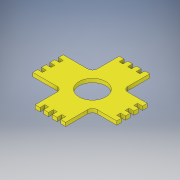
# Autodesk Inventor part: cross
Saved by Autodesk Inventor 2019.1 (Build 231200000, 200)
## iProperties
Created: 2018-10-29
Part Number: cross
Material: Generic
Document SubType Name: Modeling
Designer: kfortuna
Density: 1 g/cm^3
Appearance: Default
Author: kfortuna
Autodesk Inventor part; units mm, degrees
ref_plane "YZ Plane" through (0, 0, 0) normal (1, 0, 0) x (0, 1, 0)
ref_plane "XZ Plane" through (0, 0, 0) normal (0, 1, 0) x (-1, 0, 0)
ref_plane "XY Plane" through (0, 0, 0) normal (0, 0, 1) x (1, 0, 0)
sketch "Sketch2" plane through (0, 0, 0) normal (0, 1, 0) x (-1, 0, 0)
  line L0 (35.4299, 28.2779) -> (35.4299, 34.5151)
  line L1 (35.4299, 51.0151) -> (35.4299, 60.0151)
  line L2 (47.4299, 49.0151) -> (37.4299, 49.0151)
  line L3 (20.9299, 49.0151) -> (12.9299, 49.0151)
  line L4 (22.9299, 55.7744) -> (22.9299, 51.0151)
  line L5 (22.9299, 34.5151) -> (22.9299, 26.5151)
  line L6 (12.9299, 36.5151) -> (20.9299, 36.5151)
  line L7 (37.4299, 36.5151) -> (47.4299, 36.5151)
  line L8 (12.9299, 38.5151) -> (14.9299, 38.5151)
  line L9 (14.9299, 38.5151) -> (14.9299, 40.0151)
  line L10 (14.9299, 40.0151) -> (12.9299, 40.0151)
  line L11 (12.9299, 42.0151) -> (14.9299, 42.0151)
  line L12 (14.9299, 42.0151) -> (14.9299, 43.5151)
  line L13 (14.9299, 43.5151) -> (12.9299, 43.5151)
  line L14 (12.9299, 45.5151) -> (14.9299, 45.5151)
  line L15 (14.9299, 45.5151) -> (14.9299, 47.0151)
  line L16 (14.9299, 47.0151) -> (12.9299, 47.0151)
  line L17 (12.9299, 49.0151) -> (12.9299, 47.0151)
  line L18 (12.9299, 45.5151) -> (12.9299, 43.5151)
  line L19 (12.9299, 42.0151) -> (12.9299, 40.0151)
  line L20 (12.9299, 38.5151) -> (12.9299, 36.5151)
  line L21 (33.4299, 27.5151) -> (33.4299, 25.5151)
  line L22 (31.9299, 25.5151) -> (31.9299, 27.5151)
  line L23 (29.9299, 27.5151) -> (29.9299, 25.5151)
  line L24 (28.4299, 25.5151) -> (28.4299, 27.5151)
  line L25 (26.4299, 27.5151) -> (26.4299, 25.5151)
  line L26 (24.9299, 25.5151) -> (24.9299, 27.5151)
  line L27 (47.4299, 47.0151) -> (45.4299, 47.0151)
  line L28 (47.4299, 45.5151) -> (45.4299, 45.5151)
  line L29 (47.4299, 43.5151) -> (45.4299, 43.5151)
  line L30 (47.4299, 42.0151) -> (45.4299, 42.0151)
  line L31 (47.4299, 40.0151) -> (45.4299, 40.0151)
  line L32 (47.4299, 38.5151) -> (45.4299, 38.5151)
  line L33 (45.4299, 38.5151) -> (45.4299, 40.0151)
  line L34 (45.4299, 42.0151) -> (45.4299, 43.5151)
  line L35 (45.4299, 45.5151) -> (45.4299, 47.0151)
  line L36 (47.4299, 36.5151) -> (47.4299, 38.5151)
  line L37 (47.4299, 40.0151) -> (47.4299, 42.0151)
  line L38 (47.4299, 43.5151) -> (47.4299, 45.5151)
  line L39 (47.4299, 47.0151) -> (47.4299, 49.0151)
  line L40 (33.4299, 60.0151) -> (33.4299, 58.0151)
  line L41 (31.9299, 60.0151) -> (31.9299, 58.0151)
  line L42 (29.9299, 60.0151) -> (29.9299, 58.0151)
  line L43 (28.4299, 60.0151) -> (28.4299, 58.0151)
  line L44 (26.4299, 60.0151) -> (26.4299, 58.0151)
  line L45 (24.9299, 60.0151) -> (24.9299, 58.0151)
  arc A0 (35.4299, 51.0151) -> (37.4299, 49.0151) centre (37.4299, 51.0151) ccw
  arc A1 (37.4299, 36.5151) -> (35.4299, 34.5151) centre (37.4299, 34.5151) ccw
  arc A2 (22.9299, 34.5151) -> (20.9299, 36.5151) centre (20.9299, 34.5151) ccw
  arc A3 (20.9299, 49.0151) -> (22.9299, 51.0151) centre (20.9299, 51.0151) ccw
  line L46 (35.4299, 28.2779) -> (35.4299, 25.5151)
  line L47 (22.9299, 26.5151) -> (22.9299, 25.5151)
  line L48 (35.4299, 25.5151) -> (33.4299, 25.5151)
  line L49 (31.9299, 25.5151) -> (29.9299, 25.5151)
  line L50 (28.4299, 25.5151) -> (26.4299, 25.5151)
  line L51 (24.9299, 25.5151) -> (22.9299, 25.5151)
  line L52 (24.9299, 27.5151) -> (26.4299, 27.5151)
  line L53 (28.4299, 27.5151) -> (29.9299, 27.5151)
  line L54 (31.9299, 27.5151) -> (33.4299, 27.5151)
  line L55 (22.9299, 55.7744) -> (22.9299, 60.0151)
  line L56 (35.4299, 60.0151) -> (33.4299, 60.0151)
  line L57 (31.9299, 60.0151) -> (29.9299, 60.0151)
  line L58 (28.4299, 60.0151) -> (26.4299, 60.0151)
  line L59 (24.9299, 60.0151) -> (22.9299, 60.0151)
  line L60 (24.9299, 58.0151) -> (26.4299, 58.0151)
  line L61 (28.4299, 58.0151) -> (29.9299, 58.0151)
  line L62 (31.9299, 58.0151) -> (33.4299, 58.0151)
  circle A4 centre (29.1799, 42.7651) radius 5.5
  point P0 (0, 0)
  point P1 (35.4299, 36.5151)
  point P2 (35.4299, 49.0151)
  point P3 (22.9299, 49.0151)
  point P4 (22.9299, 36.5151)
  dimension "d25" = 1.5
  dimension "d26" = 1.5
  dimension "d27" = 1.5
  dimension "d28" = 2
  dimension "d29" = 2
  dimension "d30" = 2
  dimension "d31" = 2
  dimension "d43" = 2
  dimension "d44" = 2
  dimension "d45" = 2
  dimension "d46" = 2
  dimension "d47" = 2
  dimension "d48" = 2
  dimension "d49" = 2
  dimension "d50" = 2
  dimension "d51" = 2
  dimension "d52" = 2
  dimension "d53" = 2
  dimension "d60" = 2
  dimension "d61" = 1.5
  dimension "d62" = 1.5
  dimension "d63" = 1.5
  dimension "d64" = 1.5
  dimension "d65" = 1.5
  dimension "d66" = 1.5
  dimension "d67" = 1.5
  dimension "d68" = 1.5
  dimension "d69" = 1.5
  dimension "d70" = 2
  dimension "d71" = 2
  dimension "d72" = 2
  dimension "d74" = 2
  dimension "d75" = 2
  dimension "d76" = 2
  dimension "d77" = 2
  dimension "d78" = 2
  dimension "d79" = 2
  dimension "d80" = 2
  dimension "d81" = 11
  dimension "d82" = 11
  dimension "d83" = 11
  dimension "d84" = 11
  dimension "d85" = 2
  dimension "d86" = 2
  dimension "d87" = 2
  dimension "d88" = 2
  dimension "d89" = 10
  dimension "d90" = 10
  dimension "d91" = 12
  dimension "d92" = 12
  dimension "d97" = 2
  dimension "d98" = 2
  dimension "d99" = 2
  dimension "d100" = 8
  dimension "d102" = 2
  dimension "d105" = 6.25
  dimension "d106" = 6.25
  dimension "d109" = 2
  dimension "d110" = 0
  dimension "d111" = 2
  dimension "d112" = 0
  dimension "d113" = 2
  constraints: 126 end point, 31 parallel, 28 perpendicular, 12 horizontal, 12 point on line, 10 collinear, 8 point on circle, 8 tangent, 6 vertical, 5 centre point, 3 equal radius
  measures "d25" distance of L8.end L9.end
  measures "d26" distance of L11.end L12.end
  measures "d27" distance of L14.end L15.end
  measures "d28" distance between parallel lines of L16 L3
  measures "d29" distance between parallel lines of L13 L14
  measures "d30" distance between parallel lines of L10 L11
  measures "d31" distance between parallel lines of L6 L8
  measures "d43" distance of L8.start L8.end
  measures "d44" distance of L9.end L10.end
  measures "d45" distance of L12.end L13.end
  measures "d46" distance of L15.end L16.end
  measures "d47" distance of L32.start L32.end
  measures "d48" distance of L31.start L31.end
  measures "d49" distance of L30.start L30.end
  measures "d50" distance of L29.start L29.end
  measures "d51" distance of L28.start L28.end
  measures "d52" distance of L27.start L27.end
  measures "d53" distance from line of L27.end L2
  measures "d60" radius of A0
  measures "d61" distance of L22.end L21.start
  measures "d62" distance of L24.end L23.start
  measures "d63" distance of L26.end L25.start
  measures "d64" distance of L32.end L31.end
  measures "d65" distance of L30.end L29.end
  measures "d66" distance of L28.end L27.end
  measures "d67" distance of L41.end L40.end
  measures "d68" distance of L43.end L42.end
  measures "d69" distance of L45.end L44.end
  measures "d70" distance of L7.end L32.start
  measures "d71" distance of L31.start L30.start
  measures "d72" distance of L29.start L28.start
  measures "d74" distance of L41.start L42.start
  measures "d75" distance of L43.start L44.start
  measures "d76" distance of L45.start L55.end
  measures "d77" distance of L46.end L21.end
  measures "d78" distance of L22.start L23.end
  measures "d79" distance of L24.start L25.end
  measures "d80" distance of L26.start L47.end
  measures "d81" distance between parallel lines of L7 L48
  measures "d82" distance between parallel lines of L51 L6
  measures "d83" distance between parallel lines of L59 L3
  measures "d84" distance between parallel lines of L56 L2
  measures "d85" distance between parallel lines of L54 L48
  measures "d86" distance of L23.start L23.end
  measures "d87" distance of L24.start L24.end
  measures "d88" distance of L25.start L25.end
  measures "d89" distance between parallel lines of L20 L5
  measures "d90" distance between parallel lines of L17 L4
  measures "d91" distance between parallel lines of L1 L39
  measures "d92" distance between parallel lines of L0 L36
  measures "d97" distance between parallel lines of L53 L49
  measures "d98" distance between parallel lines of L50 L52
  measures "d99" distance between parallel lines of L51 L52
  measures "d100" distance of L5.start L5.end
  measures "d102" distance between parallel lines of L1 L40
  measures "d105" horizontal distance of A4.centre point (35.43, 36.515)
  measures "d106" horizontal distance of point (22.93, 49.015) A4.centre
  measures "d109" distance of L40.start L40.end
  measures "d110" distance between parallel lines of L56 L57
  measures "d111" distance between parallel lines of L57 L61
  measures "d112" distance between parallel lines of L57 L58
  measures "d113" distance between parallel lines of L60 L58
extrude "Extrusion3" add sketch "Sketch2" along normal blind 1.524
body "Solid3"
